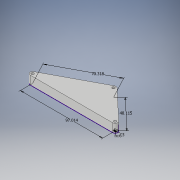
# Autodesk Inventor part: ternary_link
Saved by Autodesk Inventor 2019 (Build 230136000, 136)
## iProperties
Created: 2021-02-18
Part Number: ternary_link
Material: 一般
Document SubType Name: Modeling
Designer: wasd5
Density: 1 g/cm^3
Appearance: 預設
Author: wasd5
Autodesk Inventor part; units mm, degrees
ref_plane "YZ Plane" through (0, 0, 0) normal (1, 0, 0) x (0, 1, 0)
ref_plane "XZ Plane" through (0, 0, 0) normal (0, 1, 0) x (-1, 0, 0)
ref_plane "XY Plane" through (0, 0, 0) normal (0, 0, 1) x (1, 0, 0)
sketch "草圖2" plane through (0, 0, 0) normal (0, 1, 0) x (-1, 0, 0)
  line L0 (-62.0601, -33.0641) -> (0, 0) construction
  line L1 (0, 0) -> (-97.0141, 0) construction
  arc A0 (-97.0141, 3) -> (-99.0756, -2.1794) centre (-97.0141, 0) ccw
  arc A1 (1.4106, -2.6477) -> (0, 3) centre (0, 0) ccw
  line L2 (-97.0141, 3) -> (0, 3)
  line L3 (-99.0756, -2.1794) -> (-64.1217, -35.2435)
  line L4 (-97.0141, 0) -> (-62.0601, -33.0641) construction
  arc A2 (-64.1217, -35.2435) -> (-60.6495, -35.7117) centre (-62.0601, -33.0641) ccw
  line L5 (1.4106, -2.6477) -> (-60.6495, -35.7117)
  circle A3 centre (-97.0141, 0) radius 1.5
  circle A4 centre (0, 0) radius 1.5
  circle A5 centre (-62.0601, -33.0641) radius 1.5
  dimension "d11" = 6
  dimension "hole" = 3
  dimension "center_distance1" = 97.0141
  dimension "center_distance3" = 48.1146
  dimension "center_distance2" = 70.3185
  constraints: 12 end point, 7 coincident, 6 centre point, 6 point on circle, 6 tangent, 4 equal radius, 1 horizontal
  measures "d11" diameter of A0
  measures "hole" diameter of A3
  measures "center_distance1" distance of L1.start L1.end
  measures "center_distance3" distance of L4.start L4.end
  measures "center_distance2" distance of L4.end L1.start
extrude "擠出2" add sketch "草圖2" along normal blind 10
equation "\"d11\" = 2 * hole"
